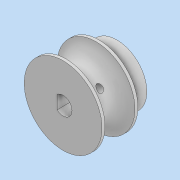
# Autodesk Inventor part: 지름 핸들러
Saved by Autodesk Inventor 2020 (Build 240168000, 168)
## iProperties
Created: 2020-05-05
Part Number: 지름 핸들러
Material: 일반
Document SubType Name: Modeling
Designer: sbahn
Density: 1 g/cm^3
Appearance: 기본값
Author: sbahn
Autodesk Inventor part; units mm, degrees
ref_plane "YZ Plane" through (0, 0, 0) normal (1, 0, 0) x (0, 1, 0)
ref_plane "XZ Plane" through (0, 0, 0) normal (0, 1, 0) x (-1, 0, 0)
ref_plane "XY Plane" through (0, 0, 0) normal (0, 0, 1) x (1, 0, 0)
sketch "스케치1" plane through (0, 0, 0) normal (1, 0, 0) x (0, 1, 0)
  line L0 (0, 0) -> (0, -9)
  line L1 (0, 0) -> (1.5, 0)
  line L2 (1.5, 0) -> (1.5, -9)
  line L3 (1.5, -9) -> (5, -9)
  line L4 (5, -9) -> (5, -6)
  line L5 (5, -6) -> (6.5, -6)
  line L6 (1.5, 0) -> (6.5, 0)
  line L7 (6.5, 0) -> (6.5, -0.5)
  line L8 (6.5, -3) -> (1.5, -3) construction
  line L9 (6.5, -6) -> (6.5, -5.5)
  arc A0 (6.5, -0.5) -> (6.5, -5.5) centre (6.5, -3) ccw
  dimension "d0" = 9
  dimension "d2" = 9
  dimension "d3" = 3
  dimension "d4" = 10
  dimension "d6" = 3
  dimension "d7" = 3
  dimension "d8" = 13
  dimension "d9" = 0.5
  dimension "d10" = 0.5
  dimension "d11" = 13
  constraints: 20 end point, 6 perpendicular, 2 horizontal, 2 point on circle, 2 vertical, 1 centre point, 1 coincident, 1 point on line
  measures "d0" distance of L0.start L0.end
  measures "d2" distance between parallel lines of L6 L3
  measures "d3" diameter of L2 L0
  measures "d4" diameter of L4 L0
  measures "d6" distance of L3.end L4.end
  measures "d7" distance between parallel lines of L6 L8
  measures "d8" diameter of L7 L0
  measures "d9" distance of L5.end L9.end
  measures "d10" distance of L6.end L7.end
  measures "d11" diameter of L8.start L0
revolve "회전1" add sketch "스케치1" angle 360 about axis through (0, 0, 0) along (0, 0, -1)
sketch "스케치2" plane through (0, 0, -9) normal (0, 0, -1) x (-1, 0, 0)
  circle A0 centre (0, 0) radius 1.5 projected
  line L0 (1, 1.118) -> (1, -1.118)
  dimension "d13" = 1
  constraints: 2 end point, 2 point on circle, 1 vertical
  measures "d13" distance from line of point (0, 0) L0
extrude "돌출1" add sketch "스케치2" against normal blind 9 contours A0 L0 picked at (1.1667, 0)
ref_plane "작업 평면1" through (0, 0, -3) normal (0, 0, 1) x (1, 0, 0)
sketch "스케치3" plane through (0, 0, -3) normal (0, 0, 1) x (1, 0, 0)
  line L0 (3.0429, 2.5) -> (-2.6844, 2.5)
  line L1 (-5.7069, 2.5) -> (4.2931, 2.5)
  line L2 (4.2931, 2.5) -> (4.2931, 3)
  line L3 (4.2931, 3) -> (-5.7069, 3)
  line L4 (-5.7069, 3) -> (-5.7069, 2.5)
  point P0 (0, 0)
  dimension "d16" = 0.5
  dimension "d17" = 2.5
  dimension "d18" = 10
  constraints: 10 end point, 2 horizontal, 2 parallel, 1 perpendicular, 1 point on line
  measures "d16" distance between parallel lines of L0 L3
  measures "d17" distance from line of point (0, 0) L0
  measures "d18" distance between parallel lines of L4 L2
revolve "회전2" cut sketch "스케치3" angle 360 about axis through (-5.7069, 2.5, -3) along (1, 0, 0)
